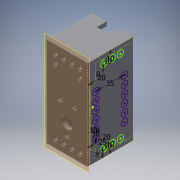
# Autodesk Inventor part: Motor cover lower
Saved by Autodesk Inventor 2019 (Build 230136000, 136)
## iProperties
Created: 2018-11-25
Part Number: Motor cover lower
Material: Generic
Document SubType Name: Modeling
Designer: Varga Daniel
Density: 1 g/cm^3
Appearance: Default
Author: Varga Daniel
Autodesk Inventor part; units mm, degrees
ref_plane "YZ Plane" through (0, 0, 0) normal (1, 0, 0) x (0, 1, 0)
ref_plane "XZ Plane" through (0, 0, 0) normal (0, 1, 0) x (-1, 0, 0)
ref_plane "XY Plane" through (0, 0, 0) normal (0, 0, 1) x (1, 0, 0)
ref_plane "Work Plane2" through (20, -5.2, 6) normal (0, 0, 1) x (1, 0, 0)
sketch "Sketch1" plane through (20, -5.2, 6) normal (0, 0, 1) x (1, 0, 0)
  line L0 (-33.75, 55) -> (16.25, 55)
  line L1 (16.25, 55) -> (16.25, -55)
  line L2 (16.25, -55) -> (-33.75, -55)
  line L3 (-33.75, -55) -> (-33.75, 55)
  line L4 (-8.75, 55) -> (-8.75, -55) construction
  circle A0 centre (-17.5, 0) radius 1.35
  circle A1 centre (0, 0) radius 1.35
  circle A2 centre (-8.75, -34.3) radius 1.35
  circle A3 centre (-8.75, -20.6) radius 7.25
  line L5 (-33.75, 0) -> (16.25, 0) construction
  point P0 (-8.75, 0)
  dimension "d0" = 50
  dimension "d1" = 110
  dimension "d15" = 2.7
  dimension "d16" = 2.7
  dimension "d17" = 2.7
  dimension "d18" = 14.5
  dimension "d19" = 17.5
  dimension "d20" = 20.6
  dimension "d21" = 34.3
  dimension "d38" = 8.75
  dimension "d49" = 55
  constraints: 12 end point, 5 midpoint, 4 centre point, 4 point on line, 2 horizontal, 2 parallel, 2 perpendicular, 1 vertical
  measures "d0" distance between parallel lines of L3 L1
  measures "d1" distance between parallel lines of L2 L0
  measures "d15" diameter of A0
  measures "d16" diameter of A1
  measures "d17" diameter of A2
  measures "d18" diameter of A3
  measures "d19" distance of A1.centre A0.centre
  measures "d20" vertical distance of A3.centre A0.centre
  measures "d21" vertical distance of A2.centre A0.centre
  measures "d38" distance from line of L4 A0.centre
  measures "d49" distance between parallel lines of L2 L5
extrude "Extrusion2" add sketch "Sketch1" against normal blind 4
sketch "Sketch2" plane through (20, -5.2, 6) normal (0, 0, 1) x (1, 0, 0)
  circle A0 centre (-8.75, -20.6) radius 7.25 construction
  circle A1 centre (-8.75, -34.3) radius 1.35 construction
  circle A2 centre (0, 0) radius 1.35 construction
  circle A3 centre (-17.5, 0) radius 1.35 construction
  line L0 (-33.75, 55) -> (16.25, 55) construction
  line L1 (-33.75, -55) -> (-33.75, 55) construction
  line L2 (16.25, -55) -> (-33.75, -55) construction
  line L3 (16.25, 55) -> (16.25, -55) construction
  line L4 (-14.4, -1.7898) -> (-17.5, -3.5796)
  line L5 (-17.5, -3.5796) -> (-20.6, -1.7898)
  line L6 (-20.6, -1.7898) -> (-20.6, 1.7898)
  line L7 (-20.6, 1.7898) -> (-17.5, 3.5796)
  line L8 (-17.5, 3.5796) -> (-14.4, 1.7898)
  line L9 (-14.4, 1.7898) -> (-14.4, -1.7898)
  line L10 (3.1, -1.7898) -> (0, -3.5796)
  line L11 (0, -3.5796) -> (-3.1, -1.7898)
  line L12 (-3.1, -1.7898) -> (-3.1, 1.7898)
  line L13 (-3.1, 1.7898) -> (0, 3.5796)
  line L14 (0, 3.5796) -> (3.1, 1.7898)
  line L15 (3.1, 1.7898) -> (3.1, -1.7898)
  line L16 (-5.65, -36.0898) -> (-8.75, -37.8796)
  line L17 (-8.75, -37.8796) -> (-11.85, -36.0898)
  line L18 (-11.85, -36.0898) -> (-11.85, -32.5102)
  line L19 (-11.85, -32.5102) -> (-8.75, -30.7204)
  line L20 (-8.75, -30.7204) -> (-5.65, -32.5102)
  line L21 (-5.65, -32.5102) -> (-5.65, -36.0898)
  line L22 (-33.75, -55) -> (-33.75, 55) projected
  point P0 (-20, 5.2)
  dimension "d26" = 6.2
  dimension "d27" = 6.2
  dimension "d28" = 6.2
  constraints: 36 end point, 3 coincident, 3 parallel, 39 other
  measures "d26" distance between parallel lines of L9 L6
  measures "d27" distance between parallel lines of L15 L12
  measures "d28" distance between parallel lines of L18 L21
extrude "Extrusion3" cut sketch "Sketch2" against normal blind 2.3
sketch "Sketch3" plane through (20, -5.2, 2) normal (0, 0, -1) x (-1, 0, 0)
  line L0 (19.7, 4.9) -> (-2.2, 4.9) construction
  line L1 (19.7, -28.8) -> (19.7, 4.9) construction
  arc A0 (17, -31.5) -> (19.7, -28.8) centre (17, -28.8) ccw construction
  line L2 (0.5, -31.5) -> (17, -31.5) construction
  arc A1 (-2.2, -28.8) -> (0.5, -31.5) centre (0.5, -28.8) ccw construction
  line L3 (-2.2, 4.9) -> (-2.2, -28.8) construction
  circle A2 centre (17.5, 0) radius 1.4 construction
  circle A3 centre (0, 0) radius 1.4 construction
  circle A4 centre (8.75, -9.4404) radius 2.05 construction
  circle A5 centre (8.85, -20.6) radius 2.8 construction
  arc A6 (-2.7, -28.8) -> (0.5, -32) centre (0.5, -28.8) ccw
  line L4 (0.5, -32) -> (17, -32)
  arc A7 (17, -32) -> (20.2, -28.8) centre (17, -28.8) ccw
  line L5 (20.2, -28.8) -> (20.2, 5.4)
  line L6 (20.2, 5.4) -> (-2.7, 5.4)
  line L7 (-2.7, 5.4) -> (-2.7, -28.8)
  circle A8 centre (0, 0) radius 1.9
  circle A9 centre (17.5, 0) radius 1.9
  circle A10 centre (8.75, -9.4404) radius 2.55
  circle A11 centre (8.75, -20.6) radius 7.25 construction
  circle A12 centre (8.75, -20.6) radius 7.75
  point P0 (20, 5.2)
  dimension "d31" = 0.5
  dimension "d32" = 0.5
  dimension "d33" = 0.5
  dimension "d34" = 0.5
  dimension "d35" = 0.5
  constraints: 8 end point, 6 centre point, 4 point on circle, 5 other
  measures "d31" distance between parallel lines of L3 L7
  measures "d32" radial gap between concentric circles of A3 A8
  measures "d33" radial gap between concentric circles of A2 A9
  measures "d34" radial gap between concentric circles of A4 A10
  measures "d35" radial gap between concentric circles of A11 A12
ref_plane "Work Plane3" through (0.3, -36.7, 0.5) normal (0, 0, 1) x (1, 0, 0)
extrude "Extrusion4" add sketch "Sketch3" along normal up to surface (1.5 mm away)
sketch "Sketch4" plane through (20, -5.2, 6) normal (0, 0, 1) x (1, 0, 0)
  circle A0 centre (-23.75, 45) radius 4
  line L0 (3.1, 1.7898) -> (3.1, -1.7898) construction
  line L1 (3.1, -1.7898) -> (0, -3.5796) construction
  line L2 (0, -3.5796) -> (-3.1, -1.7898) construction
  line L3 (-3.1, -1.7898) -> (-3.1, 1.7898) construction
  line L4 (-3.1, 1.7898) -> (0, 3.5796) construction
  line L5 (0, 3.5796) -> (3.1, 1.7898) construction
  line L6 (-14.4, 1.7898) -> (-14.4, -1.7898) construction
  line L7 (-14.4, -1.7898) -> (-17.5, -3.5796) construction
  line L8 (-17.5, -3.5796) -> (-20.6, -1.7898) construction
  line L9 (-20.6, -1.7898) -> (-20.6, 1.7898) construction
  line L10 (-20.6, 1.7898) -> (-17.5, 3.5796) construction
  line L11 (-17.5, 3.5796) -> (-14.4, 1.7898) construction
  line L12 (-5.65, -32.5102) -> (-5.65, -36.0898) construction
  line L13 (-5.65, -36.0898) -> (-8.75, -37.8796) construction
  line L14 (-8.75, -37.8796) -> (-11.85, -36.0898) construction
  line L15 (-11.85, -36.0898) -> (-11.85, -32.5102) construction
  line L16 (-11.85, -32.5102) -> (-8.75, -30.7204) construction
  line L17 (-8.75, -30.7204) -> (-5.65, -32.5102) construction
  circle A1 centre (-8.75, -20.6) radius 7.25 construction
  line L18 (-33.75, 55) -> (16.25, 55) construction
  line L19 (-33.75, -55) -> (-33.75, 55) construction
  line L20 (16.25, -55) -> (-33.75, -55) construction
  line L21 (16.25, 55) -> (16.25, -55) construction
  circle A2 centre (-13.75, 45) radius 4
  circle A3 centre (-3.75, 45) radius 4
  circle A4 centre (6.25, 45) radius 4
  circle A5 centre (-23.75, -45) radius 4
  circle A6 centre (-13.75, -45) radius 4
  circle A7 centre (-3.75, -45) radius 4
  circle A8 centre (6.25, -45) radius 4
  circle A9 centre (-23.75, 35) radius 4
  circle A10 centre (6.25, 35) radius 4
  point P0 (-20, 5.2)
  dimension "d39" = 8
  dimension "d40" = 10
  dimension "d41" = 10
  dimension "d44" = 10
  dimension "d50" = 8
  dimension "d51" = 10
  dimension "d52" = 10
  dimension "d58" = 10
  dimension "d80" = 10
  dimension "d87" = 10
  constraints: 10 centre point, 2 horizontal, 2 vertical, 16 other
  measures "d39" diameter of A0
  measures "d40" distance from line of A0.centre L19
  measures "d41" distance from line of A0.centre L18
  measures "d44" distance of A0.centre A2.centre
  measures "d50" diameter of A5
  measures "d51" distance from line of A5.centre L19
  measures "d52" distance from line of A5.centre L20
  measures "d58" distance of A5.centre A6.centre
  measures "d80" distance of A0.centre A9.centre
  measures "d87" distance of A4.centre A10.centre
extrude "Extrusion5" cut sketch "Sketch4" against normal blind 0.8
sketch "Sketch5" plane through (16.25, 39.8, 5.2) normal (0, 0, 1) x (1, 0, 0)
  circle A0 centre (0, -90) radius 4 construction
  circle A1 centre (-20, -90) radius 4 construction
  circle A2 centre (0, 0) radius 4 construction
  circle A3 centre (-20, 0) radius 4 construction
  circle A4 centre (-10, 0) radius 4 construction
  circle A5 centre (10, 0) radius 4 construction
  circle A6 centre (-10, -90) radius 4 construction
  circle A7 centre (10, -90) radius 4 construction
  line L0 (6.85, -43.2102) -> (6.85, -46.7898) construction
  line L1 (6.85, -46.7898) -> (3.75, -48.5796) construction
  line L2 (3.75, -48.5796) -> (0.65, -46.7898) construction
  line L3 (0.65, -46.7898) -> (0.65, -43.2102) construction
  line L4 (0.65, -43.2102) -> (3.75, -41.4204) construction
  line L5 (3.75, -41.4204) -> (6.85, -43.2102) construction
  line L6 (-10.65, -43.2102) -> (-10.65, -46.7898) construction
  line L7 (-10.65, -46.7898) -> (-13.75, -48.5796) construction
  line L8 (-13.75, -48.5796) -> (-16.85, -46.7898) construction
  line L9 (-16.85, -46.7898) -> (-16.85, -43.2102) construction
  line L10 (-16.85, -43.2102) -> (-13.75, -41.4204) construction
  line L11 (-13.75, -41.4204) -> (-10.65, -43.2102) construction
  line L12 (-1.9, -77.5102) -> (-1.9, -81.0898) construction
  line L13 (-1.9, -81.0898) -> (-5, -82.8796) construction
  line L14 (-5, -82.8796) -> (-8.1, -81.0898) construction
  line L15 (-8.1, -81.0898) -> (-8.1, -77.5102) construction
  line L16 (-8.1, -77.5102) -> (-5, -75.7204) construction
  line L17 (-5, -75.7204) -> (-1.9, -77.5102) construction
  circle A8 centre (-5, -65.6) radius 7.25 construction
  line L18 (-30, 10) -> (20, 10) construction
  line L19 (-30, -100) -> (-30, 10) construction
  line L20 (20, -100) -> (-30, -100) construction
  line L21 (20, 10) -> (20, -100) construction
  circle A9 centre (10, -10) radius 4 construction
  circle A10 centre (-20, -10) radius 4 construction
  point P0 (-16.25, -39.8)
sketch "Sketch6" plane through (20, -5.2, 2) normal (0, 0, -1) x (-1, 0, 0)
  circle A0 centre (3.75, -45) radius 4 construction
  circle A1 centre (23.75, -45) radius 4 construction
  circle A2 centre (3.75, 45) radius 4 construction
  circle A3 centre (23.75, 45) radius 4 construction
  circle A4 centre (13.75, 45) radius 4 construction
  circle A5 centre (-6.25, 45) radius 4 construction
  circle A6 centre (13.75, -45) radius 4 construction
  circle A7 centre (-6.25, -45) radius 4 construction
  line L0 (-3.1, 1.7898) -> (-3.1, -1.7898) construction
  line L1 (-3.1, -1.7898) -> (0, -3.5796) construction
  line L2 (0, -3.5796) -> (3.1, -1.7898) construction
  line L3 (3.1, -1.7898) -> (3.1, 1.7898) construction
  line L4 (3.1, 1.7898) -> (0, 3.5796) construction
  line L5 (0, 3.5796) -> (-3.1, 1.7898) construction
  line L6 (14.4, 1.7898) -> (14.4, -1.7898) construction
  line L7 (14.4, -1.7898) -> (17.5, -3.5796) construction
  line L8 (17.5, -3.5796) -> (20.6, -1.7898) construction
  line L9 (20.6, -1.7898) -> (20.6, 1.7898) construction
  line L10 (20.6, 1.7898) -> (17.5, 3.5796) construction
  line L11 (17.5, 3.5796) -> (14.4, 1.7898) construction
  line L12 (5.65, -32.5102) -> (5.65, -36.0898) construction
  line L13 (5.65, -36.0898) -> (8.75, -37.8796) construction
  line L14 (8.75, -37.8796) -> (11.85, -36.0898) construction
  line L15 (11.85, -36.0898) -> (11.85, -32.5102) construction
  line L16 (11.85, -32.5102) -> (8.75, -30.7204) construction
  line L17 (8.75, -30.7204) -> (5.65, -32.5102) construction
  circle A8 centre (8.75, -20.6) radius 7.25 construction
  line L18 (33.75, 55) -> (-16.25, 55) construction
  line L19 (33.75, -55) -> (33.75, 55) construction
  line L20 (-16.25, -55) -> (33.75, -55) construction
  line L21 (-16.25, 55) -> (-16.25, -55) construction
  line L22 (-11.25, -50) -> (28.75, -50)
  line L23 (28.75, -50) -> (28.75, -40)
  line L24 (28.75, -40) -> (-11.25, -40)
  line L25 (-11.25, -40) -> (-11.25, -50)
  line L26 (-6.25, -45) -> (23.75, -45) construction
  line L27 (8.75, -45) -> (8.75, -41.9729) construction
  line L28 (-11.25, 40) -> (28.75, 40)
  line L29 (28.75, 40) -> (28.75, 50)
  line L30 (28.75, 50) -> (-11.25, 50)
  line L31 (-11.25, 50) -> (-11.25, 40)
  line L32 (-6.25, 45) -> (23.75, 45) construction
  line L33 (8.75, 45) -> (8.75, 47.3618) construction
  line L34 (28.75, 40) -> (28.75, 30)
  line L35 (28.75, 30) -> (18.75, 30)
  line L36 (-11.25, 40) -> (-11.25, 30)
  line L37 (-11.25, 30) -> (-1.25, 30)
  line L38 (-1.25, 30) -> (-1.25, 40)
  line L39 (18.75, 30) -> (18.75, 40)
  point P0 (20, 5.2)
  dimension "d65" = 40
  dimension "d66" = 10
  dimension "d67" = 40
  dimension "d68" = 10
  dimension "d92" = 10
  dimension "d93" = 10
  dimension "d95" = 10
  dimension "d96" = 10
  constraints: 36 end point, 5 horizontal, 5 perpendicular, 4 parallel, 3 point on line, 2 midpoint, 2 vertical, 1 collinear, 4 other
  measures "d65" distance of L24.end L23.end
  measures "d66" distance between parallel lines of L22 L24
  measures "d67" distance of L29.end L30.end
  measures "d68" distance between parallel lines of L28 L30
  measures "d92" distance of L28.end L34.end
  measures "d93" distance of L34.end L35.end
  measures "d95" distance of L28.start L36.end
  measures "d96" distance of L36.end L37.end
extrude "Extrusion6" add sketch "Sketch6" along normal blind 5.2
hole "Hole1" at (26.25, -50.2, 5.2) at (16.25, -50.2, 5.2) at (6.25, -50.2, 5.2) at (-3.75, -50.2, 5.2) at (-3.75, 39.8, 5.2) at (6.25, 39.8, 5.2) at (16.25, 39.8, 5.2) at (26.25, 39.8, 5.2) at (-3.75, 29.8, 5.2) at (26.25, 29.8, 5.2) direction (0, 0, -1) diameter 5 end through all
sketch "Sketch7" plane through (20, -5.2, 2) normal (0, 0, -1) x (-1, 0, 0)
  circle A0 centre (3.75, 45) radius 4 construction
  line L0 (33.75, 55) -> (-16.25, 55) projected
  line L1 (33.75, -55) -> (33.75, 55) projected
  line L2 (-16.25, 55) -> (-16.25, -55) projected
  line L3 (-16.25, -55) -> (33.75, -55) projected
  line L4 (-11.25, -50) -> (-11.25, -40) construction
  line L5 (-11.25, -40) -> (28.75, -40) construction
  line L6 (28.75, -40) -> (28.75, -50) construction
  line L7 (28.75, -50) -> (-11.25, -50) construction
  line L8 (-11.25, 50) -> (28.75, 50) construction
  line L9 (28.75, 50) -> (28.75, 30) construction
  line L10 (28.75, 30) -> (18.75, 30) construction
  line L11 (18.75, 30) -> (18.75, 40) construction
  line L12 (18.75, 40) -> (-1.25, 40) construction
  line L13 (-1.25, 40) -> (-1.25, 30) construction
  line L14 (-1.25, 30) -> (-11.25, 30) construction
  line L15 (-11.25, 30) -> (-11.25, 50) construction
  line L16 (17, -32) -> (0.5, -32) construction
  arc A1 (-2.7, -28.8) -> (0.5, -32) centre (0.5, -28.8) ccw construction
  line L17 (-2.7, -28.8) -> (-2.7, 5.4) construction
  line L18 (-2.7, 5.4) -> (20.2, 5.4) construction
  line L19 (20.2, 5.4) -> (20.2, -28.8) construction
  arc A2 (17, -32) -> (20.2, -28.8) centre (17, -28.8) ccw construction
  circle A3 centre (8.75, -34.3) radius 1.35 construction
  line L20 (33.75, 55) -> (-16.25, 55) construction
  line L21 (-16.25, 55) -> (-16.25, -55) construction
  line L22 (-16.25, -55) -> (33.75, -55) construction
  line L23 (33.75, -55) -> (33.75, 55) construction
  line L24 (28.75, 50) -> (-11.25, 50) projected
  line L25 (28.75, 50) -> (-11.25, 50)
  line L26 (-11.25, 50) -> (-11.25, -50)
  line L27 (-11.25, -50) -> (28.75, -50)
  line L28 (28.75, -50) -> (28.75, 50)
  point P0 (20, 5.2)
  constraints: 8 end point, 2 parallel, 1 horizontal, 1 perpendicular
extrude "Extrusion7" add sketch "Sketch7" along normal blind 52
sketch "Sketch8" plane through (-13.75, 49.8, 6) normal (0, 1, 0) x (1, 0, 0)
  line L0 (0, 0) -> (50, 0) construction
  line L1 (50, 0) -> (50, 56) construction
  line L2 (0, 56) -> (50, 56) construction
  line L3 (0, 0) -> (0, 56) construction
  line L4 (50, 0) -> (0, 0) construction
  line L5 (25, 0) -> (25, 56) construction
  line L6 (5, 56) -> (45, 56) projected
  line L7 (17.5, 56) -> (32.5, 56)
  line L8 (32.5, 56) -> (32.5, 44)
  line L9 (32.5, 44) -> (17.5, 44)
  line L10 (17.5, 44) -> (17.5, 56)
  point P0 (13.75, 6)
  dimension "d99" = 15
  dimension "d100" = 12
  constraints: 10 end point, 2 midpoint, 2 parallel, 1 horizontal, 1 perpendicular, 1 point on line, 1 other
  measures "d99" distance between parallel lines of L8 L10
  measures "d100" distance between parallel lines of L9 L2
extrude "Extrusion8" cut sketch "Sketch8" against normal up to next
sketch "Sketch9" plane through (36.25, -60.2, 6) normal (1, 0, 0) x (0, 0, -1)
  line L0 (9.2, 15) -> (9.2, 5) construction
  line L1 (4, 15) -> (9.2, 15) construction
  line L2 (4, 85) -> (4, 15) construction
  line L3 (4, 85) -> (9.2, 85) construction
  line L4 (9.2, 105) -> (9.2, 85) construction
  line L5 (9.2, 105) -> (56, 105) construction
  line L6 (56, 5) -> (56, 105) construction
  line L7 (9.2, 5) -> (56, 5) construction
  circle A0 centre (10, 25) radius 4
  line L8 (0, 110) -> (0, 0) construction
  line L9 (0, 0) -> (56, 0) construction
  line L10 (56, 110) -> (56, 0) construction
  line L11 (0, 110) -> (56, 110) construction
  circle A1 centre (10, 35) radius 4
  circle A2 centre (10, 45) radius 4
  circle A3 centre (10, 55) radius 4
  circle A4 centre (10, 65) radius 4
  circle A5 centre (10, 75) radius 4
  circle A6 centre (20, 100) radius 4
  circle A7 centre (30, 100) radius 4
  circle A8 centre (40, 100) radius 4
  circle A9 centre (20, 10) radius 4
  circle A10 centre (30, 10) radius 4
  circle A11 centre (40, 10) radius 4
  point P0 (6, 60.2)
  dimension "d103" = 8
  dimension "d106" = 10
  dimension "d107" = 25
  dimension "d110" = 10
  dimension "d115" = 8
  dimension "d116" = 20
  dimension "d117" = 10
  dimension "d120" = 10
  dimension "d125" = 8
  dimension "d126" = 20
  dimension "d127" = 10
  dimension "d130" = 10
  constraints: 12 centre point, 2 horizontal, 1 vertical, 18 other
  measures "d103" diameter of A0
  measures "d106" distance from line of A0.centre L8
  measures "d107" distance from line of A0.centre L9
  measures "d110" distance of A0.centre A1.centre
  measures "d115" diameter of A6
  measures "d116" distance from line of A6.centre L8
  measures "d117" distance from line of A6.centre L11
  measures "d120" distance of A6.centre A7.centre
  measures "d125" diameter of A9
  measures "d126" distance from line of A9.centre L8
  measures "d127" distance from line of A9.centre L9
  measures "d130" distance of A9.centre A10.centre
extrude "Extrusion10" cut sketch "Sketch9" against normal blind 0.8 contours A1 | A2 | A3 | A4 | A5 | A6 | A7 | A8 | A9 | A10 | A11
sketch "Sketch10" plane through (36.25, -60.2, 6) normal (1, 0, 0) x (0, 0, -1)
  circle A0 centre (30, 10) radius 4 construction
  circle A1 centre (40, 100) radius 4 construction
  circle A2 centre (20, 100) radius 4 construction
  circle A3 centre (10, 65) radius 4 construction
  circle A4 centre (10, 45) radius 4 construction
  circle A5 centre (10, 35) radius 4 construction
  circle A6 centre (10, 55) radius 4 construction
  circle A7 centre (10, 75) radius 4 construction
  circle A8 centre (30, 100) radius 4 construction
  circle A9 centre (20, 10) radius 4 construction
  circle A10 centre (40, 10) radius 4 construction
  line L0 (0, 110) -> (0, 0) construction
  line L1 (0, 0) -> (56, 0) construction
  line L2 (56, 110) -> (56, 0) construction
  line L3 (0, 110) -> (56, 110) construction
  point P0 (6, 60.2)
sketch "Sketch11" plane through (31.25, -45.2, 2) normal (-1, 0, 0) x (0, 0, 1)
  line L0 (0, 65) -> (-12, 65)
  line L1 (-12, 65) -> (-12, 15)
  line L2 (-12, 15) -> (0, 15)
  line L3 (0, 15) -> (0, 65)
  circle A0 centre (-26, -5) radius 4 construction
  circle A1 centre (-36, 85) radius 4 construction
  circle A2 centre (-16, 85) radius 4 construction
  circle A3 centre (-6, 50) radius 4 construction
  circle A4 centre (-6, 30) radius 4 construction
  circle A5 centre (-6, 20) radius 4 construction
  circle A6 centre (-6, 40) radius 4 construction
  circle A7 centre (-6, 60) radius 4 construction
  circle A8 centre (-26, 85) radius 4 construction
  circle A9 centre (-16, -5) radius 4 construction
  circle A10 centre (-36, -5) radius 4 construction
  line L4 (4, 95) -> (4, -15) construction
  line L5 (4, -15) -> (-52, -15) construction
  line L6 (-52, 95) -> (-52, -15) construction
  line L7 (4, 95) -> (-52, 95) construction
  line L8 (-5.2, 0) -> (-5.2, -10) construction
  line L9 (0, 0) -> (-5.2, 0) construction
  line L10 (0, 70) -> (0, 0) construction
  line L11 (0, 70) -> (-5.2, 70) construction
  line L12 (-5.2, 90) -> (-5.2, 70) construction
  line L13 (-5.2, 90) -> (-52, 90) construction
  line L14 (-52, -10) -> (-52, 90) construction
  line L15 (-5.2, -10) -> (-52, -10) construction
  line L16 (-11, 90) -> (-41, 90)
  line L17 (-41, 90) -> (-41, 80)
  line L18 (-41, 80) -> (-11, 80)
  line L19 (-11, 80) -> (-11, 90)
  line L20 (-5.2, -10) -> (-52, -10) projected
  line L21 (-11, -10) -> (-41, -10)
  line L22 (-41, -10) -> (-41, 0)
  line L23 (-41, 0) -> (-11, 0)
  line L24 (-11, 0) -> (-11, -10)
  point P0 (-2, 45.2)
  dimension "d146" = 12
  dimension "d148" = 5
  dimension "d149" = 5
  dimension "d150" = 10
  dimension "d151" = 5
  dimension "d152" = 5
  dimension "d153" = 5
  dimension "d154" = 5
  dimension "d155" = 10
  constraints: 24 end point, 6 parallel, 3 horizontal, 3 perpendicular, 2 point on line, 1 collinear
  measures "d146" distance between parallel lines of L1 L3
  measures "d148" distance from line of A5.centre L2
  measures "d149" distance from line of A7.centre L0
  measures "d150" distance between parallel lines of L18 L13
  measures "d151" distance from line of A2.centre L19
  measures "d152" distance from line of A1.centre L17
  measures "d153" distance from line of A10.centre L22
  measures "d154" distance from line of A9.centre L24
  measures "d155" distance between parallel lines of L15 L23
extrude "Extrusion11" add sketch "Sketch11" along normal blind 4.2
hole "Hole2" at (36.25, -25.2, -4) at (36.25, -15.2, -4) at (36.25, -5.2, -4) at (36.25, 4.8, -4) at (36.25, 14.8, -4) at (36.25, 39.8, -14) at (36.25, 39.8, -34) at (36.25, 39.8, -24) at (36.25, -50.2, -14) at (36.25, -50.2, -24) at (36.25, -50.2, -34) direction (-1, 0, 0) diameter 5 end through all
sketch "Sketch12" plane through (-13.75, -60.2, 6) normal (-1, 0, 0) x (0, 0, 1)
  circle A0 centre (-30, 10) radius 2.5 construction
  circle A1 centre (-30, 100) radius 2.5 construction
  circle A2 centre (-20, 100) radius 2.5 construction
  circle A3 centre (-10, 65) radius 2.5 construction
  circle A4 centre (-10, 45) radius 2.5 construction
  circle A5 centre (-10, 35) radius 2.5 construction
  circle A6 centre (-10, 55) radius 2.5 construction
  circle A7 centre (-10, 75) radius 2.5 construction
  circle A8 centre (-40, 100) radius 2.5 construction
  circle A9 centre (-20, 10) radius 2.5 construction
  circle A10 centre (-40, 10) radius 2.5 construction
  line L0 (0, 0) -> (0, 110) construction
  line L1 (0, 110) -> (-56, 110) construction
  line L2 (-56, 0) -> (-56, 110) construction
  line L3 (0, 0) -> (-56, 0) construction
  circle A11 centre (-30, 10) radius 4 projected
  circle A12 centre (-40, 100) radius 4 projected
  circle A13 centre (-20, 100) radius 4 projected
  circle A14 centre (-10, 65) radius 4 projected
  circle A15 centre (-10, 45) radius 4 projected
  circle A16 centre (-10, 35) radius 4 projected
  circle A17 centre (-10, 55) radius 4 projected
  circle A18 centre (-10, 75) radius 4 projected
  circle A19 centre (-30, 100) radius 4 projected
  circle A20 centre (-20, 10) radius 4 projected
  circle A21 centre (-40, 10) radius 4 projected
  line L4 (0, 110) -> (0, 0) projected
  line L5 (0, 0) -> (-56, 0) projected
  line L6 (-56, 110) -> (-56, 0) projected
  line L7 (0, 110) -> (-56, 110) projected
  point P0 (-6, 60.2)
sketch "Sketch13" plane through (-8.75, -45.2, 2) normal (1, 0, 0) x (0, 0, -1)
  circle A0 centre (26, 85) radius 2.5 projected
  circle A1 centre (16, 85) radius 2.5 projected
  circle A2 centre (36, 85) radius 2.5 projected
  line L0 (41, 90) -> (11, 90) projected
  line L1 (41, 90) -> (41, 80) projected
  line L2 (41, 80) -> (11, 80) projected
  line L3 (11, 80) -> (11, 90) projected
  circle A3 centre (26, -5) radius 2.5 projected
  circle A4 centre (16, -5) radius 2.5 projected
  circle A5 centre (36, -5) radius 2.5 projected
  line L4 (11, -10) -> (41, -10) projected
  line L5 (11, -10) -> (11, 0) projected
  line L6 (11, 0) -> (41, 0) projected
  line L7 (41, 0) -> (41, -10) projected
  circle A6 centre (6, 50) radius 2.5 projected
  circle A7 centre (6, 30) radius 2.5 projected
  circle A8 centre (6, 20) radius 2.5 projected
  circle A9 centre (6, 40) radius 2.5 projected
  circle A10 centre (6, 60) radius 2.5 projected
  line L8 (0, 65) -> (12, 65) projected
  line L9 (12, 65) -> (12, 15) projected
  line L10 (12, 15) -> (0, 15) projected
  line L11 (0, 65) -> (0, 15) projected
  point P0 (2, 45.2)
extrude "Extrusion12" add sketch "Sketch13" along normal blind 4.2
extrude "Extrusion13" cut sketch "Sketch12" against normal blind 0.8 contours A11 | A12 | A13 | A14 | A15 | A16 | A17 | A18 | A19 | A20 | A21
chamfer "Chamfer1" distance 1 angle 45 4 edges at (-13.75, -5.2, 6) (11.25, 49.8, 6) (36.25, -5.2, 6) (11.25, -60.2, 6)
fillet "Fillet1" radius 2 4 edges at (-13.75, -60.2, -22.5) (-13.75, 49.8, -22.5) (36.25, -60.2, -22.5) (36.25, 49.8, -22.5)
equation "\"d16\" = d15"
equation "\"d17\" = d15"
equation "\"d27\" = d26"
equation "\"d28\" = d26"
equation "\"d32\" = d31"
equation "\"d33\" = d31"
equation "\"d34\" = d31"
equation "\"d35\" = d31"
equation "\"d67\" = d65"
equation "\"d68\" = d66"
body "Solid2"
